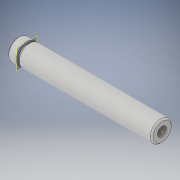
# Autodesk Inventor part: upper die center pin
Saved by Autodesk Inventor 2017 (Build 210142000, 142)
## iProperties
Created: 2017-04-14
Part Number: upper die center pin
Material: Generic
Document SubType Name: Modeling
Designer: 167942
Density: 1 g/cm^3
Appearance: Default
Author: 167942
Autodesk Inventor part; units mm, degrees
ref_plane "YZ Plane" through (0, 0, 0) normal (1, 0, 0) x (0, 1, 0)
ref_plane "XZ Plane" through (0, 0, 0) normal (0, 1, 0) x (-1, 0, 0)
ref_plane "XY Plane" through (0, 0, 0) normal (0, 0, 1) x (1, 0, 0)
sketch "Sketch1" plane through (0, 0, 0) normal (1, 0, 0) x (0, 1, 0)
  circle A0 centre (0, 0) radius 5.5563
  dimension "d0" = 11.1125
  constraints: 1 centre point, 1 coincident
  measures "d0" diameter of A0
extrude "Extrusion1" add sketch "Sketch1" along normal blind 76.2
chamfer "Chamfer1" distance 0.762 angle 45 2 edges at (76.2, -5.5563, 0) (0, -5.5563, 0)
sketch "Sketch2" plane through (76.2, 0, 0) normal (1, 0, 0) x (0, 0, -1)
  point P0 (0, 0)
sketch "Sketch3" plane through (76.2, 0, 0) normal (1, 0, 0) x (0, 0, -1)
  point P0 (0, 0)
  point P1 (0, 0)
  constraints: 1 coincident
hole "Hole1" at (76.2, 0, 0) direction (-1, 0, 0) diameter 4.9784 depth 19.05 tip angle 118 thread size "1/4-20 UNC" class "2B" standard "ANSI Unified Screw Threads"
sketch "Sketch4" plane through (0, 0, 0) normal (-1, 0, 0) x (0, 0, 1)
  point P0 (0, 0)
ref_plane "Work Plane2" through (4.7625, 0, 0) normal (-1, 0, 0) x (0, 0, 1)
sketch "Sketch5" plane through (4.7625, 0, 0) normal (-1, 0, 0) x (0, 0, 1)
  circle A0 centre (0, 0) radius 5.5562
  circle A1 centre (0, 0) radius 4.2344
  constraints: 2 centre point, 2 coincident
extrude "Extrusion2" cut sketch "Sketch5" against normal blind 1.5875
body "Solid1"
